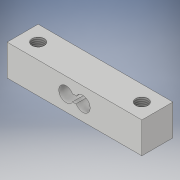
# Autodesk Inventor part: LoadCell
Saved by Autodesk Inventor 2019.3 (Build 233278000, 278)
## iProperties
Created: 2019-01-26
Part Number: LoadCell
Material: Generic
Document SubType Name: Modeling
Designer: mark
Density: 1 g/cm^3
Appearance: Default
Author: mark
Autodesk Inventor part; units mm, degrees
ref_plane "YZ Plane" through (0, 0, 0) normal (1, 0, 0) x (0, 1, 0)
ref_plane "XZ Plane" through (0, 0, 0) normal (0, 1, 0) x (-1, 0, 0)
ref_plane "XY Plane" through (0, 0, 0) normal (0, 0, 1) x (1, 0, 0)
sketch "Sketch1" plane through (0, 0, 0) normal (0, 0, 1) x (1, 0, 0)
  line L0 (0, 0) -> (55, 0)
  line L1 (55, 0) -> (55, 12.67)
  line L2 (55, 12.67) -> (0, 12.67)
  line L3 (0, 12.67) -> (0, 0)
  arc A0 (26.7926, 5.0123) -> (28.2074, 5.0123) centre (27.5, 6.335) ccw
  arc A1 (28.2074, 5.0123) -> (28.2074, 7.6577) centre (30.9, 6.335) ccw
  arc A2 (26.7926, 7.6577) -> (26.7926, 5.0123) centre (24.1, 6.335) ccw
  arc A3 (28.2074, 7.6577) -> (26.7926, 7.6577) centre (27.5, 6.335) ccw
  dimension "d0" = 55
  dimension "d1" = 12.67
  dimension "d2" = 3
  dimension "d3" = 6
  dimension "d4" = 6
  dimension "d5" = 6.8
  dimension "d6" = 6.335
  dimension "d7" = 6.335
  dimension "d9" = 6.335
  dimension "d10" = 27.5
  dimension "d11" = 3.4
  constraints: 9 point on circle, 8 end point, 4 centre point, 3 perpendicular, 1 horizontal
  measures "d0" distance of L2.end L1.end
  measures "d1" distance of L1.end L0.end
  measures "d2" diameter of A0
  measures "d3" diameter of A2
  measures "d4" diameter of A1
  measures "d5" distance of A1.centre A2.centre
  measures "d6" distance from line of L0 A2.centre
  measures "d7" distance from line of L0 A1.centre
  measures "d9" distance from line of L0 A0.centre
  measures "d10" distance from line of L3 A0.centre
  measures "d11" distance of A2.centre A0.centre
extrude "Extrusion1" add sketch "Sketch1" along normal blind 12.67
sketch "Sketch2" plane through (0, 12.67, 0) normal (0, 1, 0) x (1, 0, 0)
  circle A0 centre (6.335, -6.335) radius 2.5
  circle A1 centre (48.665, -6.335) radius 2.5
  line L0 (55, 0) -> (0, 0) projected
  line L1 (0, 0) -> (0, -12.67) projected
  line L2 (55, 0) -> (55, -12.67) projected
  dimension "d14" = 5
  dimension "d15" = 5
  dimension "d16" = 6.335
  dimension "d17" = 6.335
  dimension "d18" = 6.335
  dimension "d19" = 6.335
  constraints: 2 centre point
  measures "d14" diameter of A0
  measures "d15" diameter of A1
  measures "d16" distance from line of L0 A0.centre
  measures "d17" distance from line of L1 A0.centre
  measures "d18" distance from line of L2 A1.centre
  measures "d19" distance from line of L0 A1.centre
extrude "Extrusion2" cut sketch "Sketch2" against normal blind 12.65
thread "Thread1" size "M5x0.8" class "6H" standard "ANSI Metric M Profile" full length
thread "Thread2" size "M5x0.8" class "6H" standard "ANSI Metric M Profile" full length
body "Solid1"
